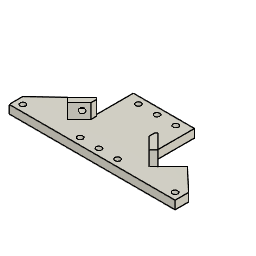
Testbed assembly v4 (Autodesk Fusion 360 archive; units mm, degrees)
design "Y axis wheel frame"
Autodesk Fusion 360 part; units mm, degrees
sketch "Sketch1" plane through (0, 0, 0) normal (0, 0, 1) x (1, 0, 0)
  line L0 (-100, 0) -> (100, 0)
  line L1 (100, 0) -> (91.75, 0) construction
  line L2 (91.75, 0) -> (91.75, 8.25) construction
  line L3 (91.75, 8.25) -> (100, 8.25) construction
  line L4 (100, 8.25) -> (100, 0) construction
  line L5 (-100, 0) -> (-91.75, 0) construction
  line L6 (-91.75, 0) -> (-91.75, 8.25) construction
  line L7 (-91.75, 8.25) -> (-100, 8.25) construction
  line L8 (-100, 8.25) -> (-100, 0) construction
  circle A0 centre (-91.75, 8.25) radius 3.25
  circle A1 centre (91.75, 8.25) radius 3.25
  line L9 (0, 0) -> (0, 60) construction
  line L10 (-48.5, 60) -> (48.5, 60) construction
  line L11 (48.5, 85) -> (60.5, 85) construction
  line L12 (60.5, 85) -> (60.5, 35) construction
  line L13 (60.5, 35) -> (48.5, 35) construction
  line L14 (48.5, 35) -> (48.5, 85) construction
  line L15 (-60.5, 85) -> (-48.5, 85) construction
  line L16 (-48.5, 85) -> (-48.5, 35) construction
  line L17 (-48.5, 35) -> (-60.5, 35) construction
  line L18 (-60.5, 35) -> (-60.5, 85) construction
  line L19 (0, 0) -> (0, 8.25) construction
  line L20 (22.5, 8.25) -> (22.5, 78.25) construction
  line L21 (22.5, 78.25) -> (-22.5, 78.25) construction
  line L22 (-22.5, 78.25) -> (-22.5, 8.25) construction
  circle A2 centre (-22.5, 78.25) radius 3.25
  circle A3 centre (22.5, 78.25) radius 3.25
  circle A4 centre (22.5, 8.25) radius 3.25
  circle A5 centre (-22.5, 8.25) radius 3.25
  line L23 (-48.5, 35) -> (-55.5711, 27.9289) construction
  line L24 (-60.5, 35) -> (-53.4289, 27.9289) construction
  line L25 (-60.5, 35) -> (-48.5, 35) construction
  line L26 (48.5, 35) -> (55.5711, 27.9289) construction
  line L27 (48.5, 35) -> (60.5, 35) construction
  line L28 (60.5, 35) -> (53.4289, 27.9289) construction
  line L29 (-54.5, 29) -> (-38.9437, 44.5563) construction
  line L30 (-54.5, 29) -> (-70.0563, 44.5563) construction
  line L31 (54.5, 29) -> (70.0563, 44.5563) construction
  line L32 (54.5, 29) -> (38.9437, 44.5563) construction
  line L33 (22.5, 8.25) -> (-22.5, 8.25) construction
  line L34 (70.0563, 44.5563) -> (72.1777, 42.435) construction
  line L35 (38.9437, 44.5563) -> (36.8223, 42.435) construction
  line L36 (-38.9437, 44.5563) -> (-36.8223, 42.435) construction
  line L37 (-70.0563, 44.5563) -> (-72.1777, 42.435) construction
  line L38 (72.1777, 42.435) -> (54.5, 24.7574)
  line L39 (36.8223, 42.435) -> (54.5, 24.7574)
  line L40 (-36.8223, 42.435) -> (-54.5, 24.7574)
  line L41 (-72.1777, 42.435) -> (-54.5, 24.7574)
  line L42 (-36.8223, 42.435) -> (-36.8223, 86.5)
  line L43 (36.8223, 42.435) -> (36.8223, 86.5)
  line L44 (36.8223, 86.5) -> (-36.8223, 86.5)
  line L45 (45.6612, 33.5962) -> (40.3579, 28.2929) construction
  line L46 (-45.6612, 33.5962) -> (-40.3579, 28.2929) construction
  line L47 (-40.3579, 28.2929) -> (-36.8223, 31.8284)
  line L48 (-36.8223, 31.8284) -> (-33.2868, 28.2929)
  line L49 (-33.2868, 28.2929) -> (-40.3579, 21.2218)
  line L50 (-40.3579, 21.2218) -> (-43.8934, 24.7574)
  line L51 (-43.8934, 24.7574) -> (-40.3579, 28.2929)
  line L52 (40.3579, 28.2929) -> (36.8223, 31.8284)
  line L53 (36.8223, 31.8284) -> (33.2868, 28.2929)
  line L54 (33.2868, 28.2929) -> (40.3579, 21.2218)
  line L55 (40.3579, 21.2218) -> (43.8934, 24.7574)
  line L56 (43.8934, 24.7574) -> (40.3579, 28.2929)
  line L57 (-91.75, 8.25) -> (-91.75, 16.5) construction
  line L58 (91.75, 8.25) -> (91.75, 16.5) construction
  line L59 (100, 16.5) -> (100, 0)
  line L60 (-100, 16.5) -> (-100, 0)
  line L61 (72.1777, 42.435) -> (100, 16.5)
  line L62 (-72.1777, 42.435) -> (-100, 16.5)
  line L63 (-36.8223, 42.435) -> (-31.519, 37.1317)
  line L64 (-31.519, 37.1317) -> (-49.1967, 19.4541)
  line L65 (-49.1967, 19.4541) -> (-54.5, 24.7574)
  line L66 (36.8223, 42.435) -> (31.519, 37.1317)
  line L67 (31.519, 37.1317) -> (49.1967, 19.4541)
  line L68 (49.1967, 19.4541) -> (54.5, 24.7574)
  line L69 (36.8223, 42.435) -> (36.8223, 31.8284)
  circle A6 centre (0, 8.25) radius 3.25
  circle A7 centre (0, 78.25) radius 3.25
  line L70 (-35, 43.25) -> (-10, 43.25) construction
  line L71 (-35, 40.6127) -> (-35, 33.6508)
  line L72 (10, 43.25) -> (35, 43.25) construction
  line L73 (35, 40.6127) -> (35, 33.6508)
  dimension "d2" = 200
  dimension "d3" = 8.25
  dimension "d4" = 8.25
  dimension "d5" = 8.25
  dimension "d6" = 8.25
  dimension "d7" = 6.5
  dimension "d8" = 6.5
  dimension "d9" = 60
  dimension "d10" = 97
  dimension "d11" = 12
  dimension "d12" = 50
  dimension "d13" = 12
  dimension "d14" = 50
  dimension "d15" = 8.25
  dimension "d16" = 45
  dimension "d17" = 70
  dimension "d18" = 6.5
  dimension "d19" = 6.5
  dimension "d20" = 6.5
  dimension "d21" = 6.5
  dimension "d22" = 10
  dimension "d24" = 45
  dimension "d25" = 10
  dimension "d26" = 45
  dimension "d27" = 10
  dimension "d28" = 10
  dimension "d29" = 22
  dimension "d30" = 22
  dimension "d31" = 22
  dimension "d32" = 22
  dimension "d33" = 3
  dimension "d34" = 3
  dimension "d35" = 3
  dimension "d36" = 3
  dimension "d37" = 25
  dimension "d38" = 25
  dimension "d39" = 25
  dimension "d41" = 25
  dimension "d44" = 7.5
  dimension "d45" = 7.5
  dimension "d46" = 5
  dimension "d47" = 5
  dimension "d48" = 10
  dimension "d49" = 5
  dimension "d50" = 5
  dimension "d51" = 5
  dimension "d52" = 10
  dimension "d53" = 5
  dimension "d54" = 86.5
  dimension "d57" = 8.25
  dimension "d58" = 8.25
  dimension "d69" = 7.5
  dimension "d70" = 25
  dimension "d71" = 7.5
  dimension "d72" = 25
  dimension "d85" = 6.5
  dimension "d86" = 6.5
  dimension "d87" = 25
  dimension "d88" = 25
  constraint horizontal L0
  constraint midpoint L9.start L0
  constraint horizontal L1
  constraint vertical L2
  constraint horizontal L3
  constraint vertical L4
  constraint horizontal L5
  constraint vertical L6
  constraint horizontal L7
  constraint vertical L8
  constraint coincident L6.end L7.start
  constraint coincident L2.end L3.start
  constraint coincident L9.start L19.start
  constraint perpendicular L0 L9
  constraint horizontal L10
  constraint midpoint L9.end L10
  constraint horizontal L11
  constraint vertical L12
  constraint horizontal L13
  constraint vertical L14
  constraint midpoint L10.end L14
  constraint horizontal L15
  constraint vertical L16
  constraint horizontal L17
  constraint vertical L18
  constraint midpoint L10.start L16
  constraint perpendicular L0 L19
  constraint vertical L20
  constraint horizontal L21
  constraint vertical L22
  constraint coincident L21.end L22.start
  constraint coincident L20.end L21.start
  constraint coincident L20.start A4.centre
  constraint coincident L22.end A5.centre
  constraint horizontal L25
  constraint perpendicular L23 L24
  constraint horizontal L27
  constraint perpendicular L26 L28
  constraint coincident L23 L29.start
  constraint coincident L24 L29.start
  constraint perpendicular L24 L29
  constraint perpendicular L23 L30
  constraint coincident L28 L31.start
  constraint coincident L26 L31.start
  constraint perpendicular L26 L31
  constraint perpendicular L31 L32
  constraint perpendicular L22 L33
  constraint midpoint L19.end L33
  constraint perpendicular L31 L34
  constraint perpendicular L32 L35
  constraint perpendicular L29 L36
  constraint perpendicular L30 L37
  constraint perpendicular L34 L38
  constraint perpendicular L35 L39
  constraint perpendicular L36 L40
  constraint perpendicular L37 L41
  constraint vertical L42
  constraint perpendicular L10 L43
  constraint midpoint L39 L45.start
  constraint perpendicular L39 L45
  constraint midpoint L40 L46.start
  constraint perpendicular L40 L46
  constraint perpendicular L46 L47
  constraint perpendicular L47 L48
  constraint perpendicular L48 L49
  constraint perpendicular L49 L50
  constraint perpendicular L45 L52
  constraint perpendicular L52 L53
  constraint perpendicular L53 L54
  constraint perpendicular L54 L55
  constraint perpendicular L7 L57
  constraint perpendicular L3 L58
  constraint vertical L60
  constraint vertical L59
  constraint perpendicular L40 L63
  constraint perpendicular L63 L64
  constraint perpendicular L39 L66
  constraint perpendicular L55 L67
  constraint coincident L19.end A6.centre
  constraint midpoint L21 A7.centre
  constraint perpendicular L22 L70
  constraint midpoint L22 L70
  constraint coincident L63 L71.start
  constraint coincident L64 L71.end
  constraint vertical L71
  constraint horizontal L72
  constraint midpoint L20 L72
  constraint coincident L66 L73.start
  constraint coincident L67 L73.end
  constraint vertical L73
  measures "d2" distance of L0.start L0.end
  measures "d3" distance of L0.end L1.end
  measures "d4" distance of L0.end L3.end
  measures "d5" distance of L0.start L5.end
  measures "d6" distance of L0.start L7.end
  measures "d7" diameter of A0
  measures "d8" diameter of A1
  measures "d9" distance of L9.start L9.end
  measures "d10" distance of L10.start L10.end
  measures "d11" distance of L11.start L11.end
  measures "d12" distance of L11.start L13.end
  measures "d13" distance of L15.start L15.end
  measures "d14" distance of L15.start L17.end
  measures "d15" distance of L9.start L19.end
  measures "d16" distance of L22.end L20.start
  measures "d17" distance of L22.end L21.end
  measures "d18" diameter of A2
  measures "d19" diameter of A3
  measures "d20" diameter of A4
  measures "d21" diameter of A5
  measures "d22" distance of L16.end L23.end
  measures "d24" angle of L24 L25
  measures "d25" distance of L17.end L24.end
  measures "d26" angle of L26 L27
  measures "d27" distance of L13.end L26.end
  measures "d28" distance of L12.end L28.end
  measures "d29" distance of L29.start L29.end
  measures "d30" distance of L29.start L30.end
  measures "d31" distance of L31.start L31.end
  measures "d32" distance of L31.start L32.end
  measures "d33" distance of L31.end L34.end
  measures "d34" distance of L32.end L35.end
  measures "d35" distance of L29.end L36.end
  measures "d36" distance of L30.end L37.end
  measures "d37" distance of L34.end L38.end
  measures "d38" distance of L35.end L38.end
  measures "d39" distance of L36.end L40.end
  measures "d41" distance of L37.end L40.end
  measures "d44" distance of L45.start L45.end
  measures "d45" distance of L46.start L46.end
  measures "d46" distance of L46.end L47.end
  measures "d47" distance of L47.end L48.end
  measures "d48" distance of L48.end L49.end
  measures "d49" distance of L49.end L50.end
  measures "d50" distance of L45.end L52.end
  measures "d51" distance of L52.end L53.end
  measures "d52" distance of L53.end L54.end
  measures "d53" distance of L54.end L55.end
  measures "d54" distance of L0 L44
  measures "d57" distance of L6.end L57.end
  measures "d58" distance of L2.end L58.end
  measures "d69" distance of L36.end L63.end
  measures "d70" distance of L63.end L64.end
  measures "d71" distance of L35.end L66.end
  measures "d72" distance of L66.end L67.end
  measures "d85" diameter of A6
  measures "d86" diameter of A7
  measures "d87" distance of L70.start L70.end
  measures "d88" distance of L72.start L72.end
extrude "Extrude2" add sketch "Sketch1" along normal blind 10 contours L0 L38 L41 L42 L43 L44 L48 L49 L50 L53 L54 L55 L59 L60 L61 L62 L63 L64 L65 L66 L67 L68 | L40 L47 L51 L63 L64 L65 L71 | L66 L67 L69 L73 | L63 L64 L71 | L47 L48 L49 L50 L51 L64 | L66 L67 L73 | L52 L53 L54 L55 L56 L67
extrude "Extrude3" add sketch "Sketch1" along normal blind 27.45 contours L40 L47 L51 L63 L64 L65 L71 | L39 L52 L56 L67 L68 L69 | L66 L67 L69 L73
sketch "Sketch4" plane through (39.6287, 39.6287, 0) normal (0.707107, 0.707107, 0) x (-0.707107, 0.707107, 0)
  line L0 (-21.0312, 0) -> (3.9688, 0)
  line L1 (3.9688, 27.45) -> (-21.0312, 27.45)
  line L2 (-21.0312, 27.45) -> (-21.0312, 10)
  line L3 (-21.0312, 10) -> (-21.0312, 0)
  line L4 (-8.5312, 27.45) -> (-8.5312, 19.2) construction
  line L5 (3.9688, 0) -> (3.9688, 10)
  line L6 (3.9688, 10) -> (3.9688, 27.45)
  dimension "d77" = 8.25
  constraint midpoint L1 L4.start
  constraint perpendicular L1 L4
  measures "d77" distance of L4.start L4.end
sketch "Sketch5" plane through (-39.6287, 39.6287, 0) normal (-0.707107, 0.707107, 0) x (-0.707107, -0.707107, 0)
  line L0 (-3.9688, 0) -> (21.0312, 0)
  line L1 (21.0312, 0) -> (21.0312, 10)
  line L2 (21.0312, 10) -> (21.0312, 27.45)
  line L3 (21.0312, 27.45) -> (-3.9688, 27.45)
  line L4 (8.5312, 27.45) -> (8.5312, 19.2) construction
  line L5 (-3.9688, 10) -> (-3.9688, 0)
  line L6 (-3.9688, 27.45) -> (-3.9688, 10)
  dimension "d78" = 8.25
  constraint midpoint L3 L4.start
  constraint perpendicular L3 L4
  measures "d78" distance of L4.start L4.end
hole "Hole3" at (-45.6612, 33.5962, 19.2) direction (0.707107, -0.707107, 0) diameter 6.5 depth 7.5 tip angle 180
hole "Hole4" at (45.6612, 33.5962, 19.2) direction (-0.707107, -0.707107, 0) diameter 6.5 depth 7.5 tip angle 180
equation "d3 = 5 mm + 3.25 mm"
equation "d4 = 5 mm + 3.25 mm"
equation "d5 = 5 mm + 3.25 mm"
equation "d6 = 5 mm + 3.25 mm"
equation "d10 = 121 mm - 24 mm"
equation "d15 = 5 mm + 3.25 mm"
equation "d54 = 90 mm - 3.5 mm"
equation "d75 = 30.7 mm - 3.25 mm"
